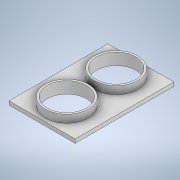
# Autodesk Inventor part: rinsing_station
Saved by Autodesk Inventor 2022 (Build 260153000, 153)
## iProperties
Created: 2022-05-04
Part Number: rinsing_station
Material: Generic
Document SubType Name: Modeling
Designer: cgbis
Density: 1 g/cm^3
Appearance: Default
Author: cgbis
Autodesk Inventor part; units mm, degrees
ref_plane "YZ Plane" through (0, 0, 0) normal (1, 0, 0) x (0, 1, 0)
ref_plane "XZ Plane" through (0, 0, 0) normal (0, 1, 0) x (-1, 0, 0)
ref_plane "XY Plane" through (0, 0, 0) normal (0, 0, 1) x (1, 0, 0)
sketch "Sketch1" plane through (0, 0, 0) normal (0, 1, 0) x (-1, 0, 0)
  point P0 (0, 0)
sketch "Sketch2" plane through (0, 0, 0) normal (0, 1, 0) x (-1, 0, 0)
  line L0 (0, 0) -> (85.5, 0)
  line L1 (85.5, 0) -> (85.5, -127.8)
  line L2 (85.5, -127.8) -> (0, -127.8)
  line L3 (0, -127.8) -> (0, 0)
  dimension "d0" = 85.5
  dimension "d1" = 127.8
  constraints: 8 end point, 2 parallel, 1 horizontal, 1 perpendicular
  measures "d0" distance of L1.end L2.end
  measures "d1" distance of L0.end L1.end
extrude "Extrusion1" add sketch "Sketch2" along normal blind 5
sketch "Sketch3" plane through (0, 5, 0) normal (0, 1, 0) x (1, 0, 0)
  line L0 (-85.5, 127.8) -> (-85.5, 0) projected
  line L1 (-85.5, 0) -> (0, 0)
  line L2 (0, 0) -> (0, 127.8)
  line L3 (0, 127.8) -> (-85.5, 127.8)
  line L4 (-85.5, 127.8) -> (-85.5, 0)
  line L5 (-2.4, 2.4) -> (-83.1, 2.4)
  line L6 (-83.1, 2.4) -> (-83.1, 125.4)
  line L7 (-83.1, 125.4) -> (-2.4, 125.4)
  line L8 (-2.4, 125.4) -> (-2.4, 2.4)
  dimension "d6" = 80.7
  dimension "d7" = 123
  constraints: 16 end point, 4 parallel, 2 horizontal, 2 perpendicular
  measures "d6" distance of L6.end L7.end
  measures "d7" distance of L5.end L6.end
extrude "Extrusion2" add sketch "Sketch3" along normal blind 120
sketch "Sketch4" plane through (0, 0, 0) normal (1, 0, 0) x (0, 0, -1)
  line L0 (10, 10) -> (117.8, 10)
  line L1 (117.8, 10) -> (117.8, 115)
  line L2 (117.8, 115) -> (10, 115)
  line L3 (10, 115) -> (10, 10)
  point P0 (0, 0)
  dimension "d10" = 107.8
  dimension "d11" = 105
  constraints: 8 end point, 2 parallel, 1 horizontal, 1 perpendicular
  measures "d10" distance of L2.end L1.end
  measures "d11" distance of L1.end L0.end
extrude "Extrusion3" cut sketch "Sketch4" against normal blind 500
sketch "Sketch5" plane through (0, 0, -127.8) normal (0, 0, -1) x (-1, 0, 0)
  line L0 (10, 10) -> (75.5, 10)
  line L1 (75.5, 10) -> (75.5, 115)
  line L2 (75.5, 115) -> (10, 115)
  line L3 (10, 115) -> (10, 10)
  point P0 (0, 0)
  dimension "d14" = 65.5
  dimension "d15" = 105
  constraints: 8 end point, 2 parallel, 1 horizontal, 1 perpendicular
  measures "d14" distance of L2.end L1.end
  measures "d15" distance of L1.end L0.end
extrude "Extrusion4" cut sketch "Sketch5" against normal blind 500
sketch "Sketch6" plane through (-85.5, 0, -127.8) normal (-1, 0, 0) x (0, 0, 1)
  line L0 (2.4, 125) -> (125.4, 125) projected
  line L1 (63.9, 125) -> (63.9, 0)
  line L2 (0, 0) -> (127.8, 0) projected
  line L3 (63.9, 125) -> (58.9, 125)
  line L4 (58.9, 125) -> (58.9, 0)
  line L5 (58.9, 0) -> (63.9, 0)
  line L6 (63.9, 0) -> (63.9, 125)
  line L7 (63.9, 125) -> (68.9, 125)
  line L8 (68.9, 125) -> (68.9, 0)
  line L9 (68.9, 0) -> (63.9, 0)
  line L10 (63.9, 0) -> (63.9, 125)
  dimension "d18" = 5
  dimension "d19" = 5
  constraints: 18 end point, 4 parallel, 2 horizontal, 2 midpoint, 2 perpendicular, 2 point on line
  measures "d18" distance of L5.end L4.end
  measures "d19" distance of L8.end L9.end
extrude "Extrusion5" add sketch "Sketch6" against normal blind 2.4
sketch "Sketch7" plane through (0, 0, 0) normal (1, 0, 0) x (0, 0, -1)
  line L0 (117.8, 115) -> (10, 115) projected
  line L1 (63.9, 115) -> (63.9, 10)
  line L2 (10, 10) -> (117.8, 10) projected
  line L3 (58.9, 10) -> (58.9, 115) projected
  line L4 (117.8, 10) -> (68.9, 10) projected
  line L5 (58.9, 115) -> (68.9, 115)
  line L6 (68.9, 115) -> (68.9, 10)
  line L7 (68.9, 10) -> (58.9, 10)
  line L8 (58.9, 10) -> (58.9, 115)
  point P0 (0, 0)
  constraints: 10 end point, 2 midpoint, 2 parallel, 1 horizontal, 1 perpendicular
extrude "Extrusion6" add sketch "Sketch7" against normal blind 2.4
sketch "Sketch8" plane through (0, 0, -127.8) normal (0, 0, -1) x (-1, 0, 0)
  line L0 (10, 100) -> (25, 115)
  line L1 (10, 115) -> (75.5, 115) projected
  line L2 (10, 100) -> (31.2132, 100) construction
  line L3 (75.5, 100) -> (60.5, 115)
  line L4 (75.5, 100) -> (96.7132, 100) construction
  line L5 (10, 10) -> (10, 115) projected
  line L6 (10, 25) -> (25, 10)
  line L7 (10, 10) -> (75.5, 10) projected
  line L8 (10, 25) -> (31.2132, 25) construction
  line L9 (75.5, 115) -> (75.5, 10) projected
  line L10 (75.5, 25) -> (60.5, 10)
  line L11 (10, 115) -> (75.5, 115)
  line L12 (75.5, 115) -> (75.5, 10)
  line L13 (75.5, 10) -> (10, 10)
  line L14 (10, 10) -> (10, 115)
  point P0 (0, 0)
  dimension "d24" = 45
  dimension "d25" = 135
  dimension "d26" = 45
  constraints: 22 end point, 6 point on line, 4 horizontal, 3 equal length, 2 parallel, 1 perpendicular
  measures "d24" angle of L2 L0
  measures "d25" angle of L4 L3
  measures "d26" angle of L6 L8
extrude "Extrusion7" add sketch "Sketch8" against normal blind 2.4 contours L5 L1 L0 | L6 L7 L5 | L1 L9 L3 | L10 L9 L7
sketch "Sketch9" plane through (-85.5, 0, 0) normal (0, 0, 1) x (1, 0, 0)
  line L0 (10, 25) -> (10, 100) projected
  line L1 (25, 115) -> (60.5, 115) projected
  line L2 (10, 100) -> (25, 115)
  line L3 (60.5, 115) -> (75.5, 100) projected
  line L4 (25, 115) -> (60.5, 115)
  line L5 (60.5, 115) -> (75.5, 100)
  line L6 (75.5, 100) -> (75.5, 25) projected
  line L7 (75.5, 100) -> (75.5, 25)
  line L8 (75.5, 25) -> (60.5, 10)
  line L9 (25, 10) -> (60.5, 10) projected
  line L10 (10, 25) -> (25, 10) projected
  line L11 (25, 10) -> (10, 25)
  line L12 (10, 25) -> (10, 100)
  line L13 (10, 115) -> (75.5, 115)
  line L14 (75.5, 115) -> (75.5, 10)
  line L15 (75.5, 10) -> (10, 10)
  line L16 (10, 10) -> (10, 115)
  point P0 (85.5, 0)
  point P1 (60.5, 10)
  constraints: 23 end point, 7 equal length, 2 horizontal, 1 perpendicular
extrude "Extrusion8" add sketch "Sketch9" against normal blind 2.4 contours L10 L15 L16 | L16 L13 L2 | L8 L14 L15 | L13 L14 L3
sketch "Sketch10" plane through (0, 0, 0) normal (1, 0, 0) x (0, 0, -1)
  line L0 (10, 115) -> (10, 10) projected
  line L1 (10, 100) -> (25, 115)
  line L2 (58.9, 115) -> (10, 115) projected
  line L3 (10, 100) -> (31.2132, 100) construction
  line L4 (58.9, 10) -> (58.9, 115) projected
  line L5 (58.9, 100) -> (43.9, 115)
  line L6 (58.9, 25) -> (43.9, 10)
  line L7 (10, 10) -> (58.9, 10) projected
  line L8 (10, 25) -> (25, 10)
  line L9 (68.9, 100) -> (83.9, 115)
  line L10 (68.9, 115) -> (117.8, 115) projected
  line L11 (68.9, 100) -> (90.1132, 100) construction
  line L12 (117.8, 115) -> (117.8, 10) projected
  line L13 (117.8, 100) -> (102.8, 115)
  line L14 (117.8, 25) -> (102.8, 10)
  line L15 (117.8, 10) -> (68.9, 10) projected
  line L16 (68.9, 25) -> (83.9, 10)
  line L17 (10, 115) -> (58.9, 115)
  line L18 (58.9, 115) -> (58.9, 10)
  line L19 (58.9, 10) -> (10, 10)
  line L20 (10, 10) -> (10, 115)
  line L21 (68.9, 115) -> (117.8, 115)
  line L22 (117.8, 115) -> (117.8, 10)
  line L23 (117.8, 10) -> (68.9, 10)
  line L24 (68.9, 10) -> (68.9, 115)
  point P0 (0, 0)
  dimension "d31" = 45
  dimension "d32" = 45
  constraints: 36 end point, 11 point on line, 6 perpendicular, 4 horizontal, 4 parallel, 2 equal length
  measures "d31" angle of L3 L1
  measures "d32" angle of L11 L9
extrude "Extrusion9" add sketch "Sketch10" against normal blind 2.4 contours L2 L1 L0 | L8 L7 L0 | L2 L4 L5 | L6 L4 L7 | L24 L10 L9 | L16 L15 L24 | L10 L12 L13 | L14 L12 L15
sketch "Sketch11" plane through (-85.5, 0, -127.8) normal (-1, 0, 0) x (0, 0, 1)
  line L0 (10, 100) -> (25, 115) projected
  line L1 (10, 100) -> (25, 115)
  line L2 (25, 115) -> (43.9, 115) projected
  line L3 (25, 115) -> (43.9, 115)
  line L4 (43.9, 115) -> (58.9, 100)
  line L5 (58.9, 100) -> (58.9, 25)
  line L6 (58.9, 25) -> (43.9, 10) projected
  line L7 (10, 10) -> (58.9, 10) projected
  line L8 (25, 10) -> (10, 25) projected
  line L9 (43.9, 10) -> (25, 10)
  line L10 (25, 10) -> (10, 25)
  line L11 (10, 25) -> (10, 100)
  line L12 (10, 115) -> (10, 10) projected
  line L13 (68.9, 25) -> (68.9, 100) projected
  line L14 (83.9, 115) -> (102.8, 115) projected
  line L15 (68.9, 100) -> (83.9, 115)
  line L16 (83.9, 115) -> (102.8, 115)
  line L17 (102.8, 115) -> (117.8, 100)
  line L18 (117.8, 25) -> (102.8, 10) projected
  line L19 (117.8, 100) -> (117.8, 25)
  line L20 (117.8, 25) -> (102.8, 10)
  line L21 (83.9, 10) -> (102.8, 10) projected
  line L22 (102.8, 10) -> (83.9, 10)
  line L23 (83.9, 10) -> (68.9, 25)
  line L24 (68.9, 25) -> (68.9, 100)
  line L25 (10, 115) -> (58.9, 115)
  line L26 (58.9, 115) -> (58.9, 10)
  line L27 (58.9, 10) -> (10, 10)
  line L28 (10, 10) -> (10, 115)
  line L29 (68.9, 115) -> (117.8, 115)
  line L30 (117.8, 115) -> (117.8, 10)
  line L31 (117.8, 10) -> (68.9, 10)
  line L32 (68.9, 10) -> (68.9, 115)
  point P0 (127.8, 0)
  constraints: 47 end point, 12 equal length, 8 perpendicular, 4 point on line, 2 horizontal
extrude "Extrusion10" add sketch "Sketch11" against normal blind 2.4 contours L12 L25 L0 | L8 L7 L12 | L25 L26 L4 | L6 L26 L7 | L23 L31 L32 | L32 L29 L15 | L18 L30 L31 | L29 L30 L17
sketch "Sketch12" plane through (0, 125, 0) normal (0, 1, 0) x (1, 0, 0)
  line L0 (-83.1, 125.4) -> (-2.4, 125.4) projected
  line L1 (-83.1, 125.4) -> (-83.1, 2.4) projected
  line L2 (-2.4, 125.4) -> (-83.1, 125.4)
  line L3 (-83.1, 125.4) -> (-83.1, 2.4)
  line L4 (-83.1, 2.4) -> (-2.4, 2.4)
  line L5 (-2.4, 2.4) -> (-2.4, 125.4)
  point P0 (0, 0)
  constraints: 8 end point, 2 parallel, 1 horizontal, 1 perpendicular
extrude "Extrusion11" add sketch "Sketch12" against normal blind 4.8
sketch "Sketch13" plane through (0, 125, 0) normal (0, 1, 0) x (1, 0, 0)
  line L0 (-2.4, 2.4) -> (-2.4, 125.4) projected
  line L1 (-83.1, 125.4) -> (-83.1, 2.4) projected
  line L2 (-2.4, 125.4) -> (-83.1, 125.4)
  line L3 (-83.1, 125.4) -> (-83.1, 2.4)
  line L4 (-83.1, 2.4) -> (-2.4, 2.4)
  line L5 (-2.4, 2.4) -> (-2.4, 125.4)
  point P0 (0, 0)
  constraints: 8 end point, 2 parallel, 1 horizontal, 1 perpendicular
extrude "Extrusion12" cut sketch "Sketch13" against normal blind 2.4
sketch "Sketch14" plane through (0, 122.6, 0) normal (0, 1, 0) x (1, 0, 0)
  line L0 (-80.1, 122.4) -> (-5.4, 122.4)
  line L1 (-5.4, 122.4) -> (-5.4, 5.4)
  line L2 (-5.4, 5.4) -> (-80.1, 5.4)
  line L3 (-80.1, 5.4) -> (-80.1, 122.4)
  point P0 (0, 0)
  dimension "d41" = 74.7
  dimension "d42" = 117
  constraints: 8 end point, 2 parallel, 1 horizontal, 1 perpendicular
  measures "d41" distance of L1.end L2.end
  measures "d42" distance of L0.end L1.end
extrude "Extrusion13" cut sketch "Sketch14" against normal blind 10
sketch "Sketch15" plane through (0, 0, 0) normal (1, 0, 0) x (0, 0, -1)
  line L0 (127.8, 0) -> (127.8, 125) projected
  line L1 (0, 125) -> (127.8, 125)
  line L2 (127.8, 125) -> (127.8, 119)
  line L3 (127.8, 119) -> (0, 119)
  line L4 (0, 119) -> (0, 125)
  line L5 (127.8, 125) -> (0, 125) projected
  line L6 (63.9, 125) -> (88.9, 125)
  line L7 (88.9, 125) -> (88.9, 119)
  line L8 (88.9, 119) -> (63.9, 119)
  line L9 (63.9, 119) -> (63.9, 125)
  line L10 (63.9, 125) -> (38.9, 125)
  line L11 (38.9, 125) -> (38.9, 119)
  line L12 (38.9, 119) -> (63.9, 119)
  line L13 (63.9, 119) -> (63.9, 125)
  point P0 (0, 0)
  dimension "d45" = 6
  dimension "d46" = 25
  dimension "d47" = 25
  constraints: 24 end point, 6 parallel, 3 horizontal, 3 perpendicular, 3 point on line, 1 midpoint
  measures "d45" distance of L1.end L2.end
  measures "d46" distance of L7.end L8.end
  measures "d47" distance of L12.end L11.end
extrude "Extrusion14" cut sketch "Sketch15" against normal blind 100 contours L3 L9 L1 L7 | L3 L11 L1 L9
sketch "Sketch16" plane through (0, 0, -127.8) normal (0, 0, -1) x (-1, 0, 0)
  line L0 (0, 125) -> (0, 119) projected
  line L1 (85.5, 0) -> (85.5, 125) projected
  line L2 (0, 125) -> (85.5, 125)
  line L3 (85.5, 125) -> (85.5, 119)
  line L4 (85.5, 119) -> (0, 119)
  line L5 (0, 119) -> (0, 125)
  line L6 (0, 125) -> (85.5, 125) projected
  line L7 (42.75, 125) -> (67.75, 125)
  line L8 (67.75, 125) -> (67.75, 119)
  line L9 (67.75, 119) -> (42.75, 119)
  line L10 (42.75, 119) -> (42.75, 125)
  line L11 (42.75, 125) -> (17.75, 125)
  line L12 (17.75, 125) -> (17.75, 119)
  line L13 (17.75, 119) -> (42.75, 119)
  line L14 (42.75, 119) -> (42.75, 125)
  point P0 (0, 0)
  dimension "d50" = 6
  dimension "d51" = 25
  dimension "d52" = 25
  constraints: 24 end point, 6 parallel, 3 horizontal, 3 perpendicular, 3 point on line, 1 midpoint
  measures "d50" distance of L2.end L3.end
  measures "d51" distance of L8.end L9.end
  measures "d52" distance of L13.end L12.end
extrude "Extrusion15" cut sketch "Sketch16" against normal blind 200 contours L2 L10 L4 L12 | L2 L8 L4 L10
sketch "Sketch17" plane through (-85.5, 0, 0) normal (0, 0, 1) x (1, 0, 0)
  line L0 (17.75, 119) -> (67.75, 119)
  line L1 (67.75, 119) -> (67.75, 118)
  line L2 (67.75, 118) -> (17.75, 118)
  line L3 (17.75, 118) -> (17.75, 119)
  point P0 (85.5, 0)
  dimension "d55" = 1
  constraints: 8 end point, 2 parallel, 1 horizontal, 1 perpendicular
  measures "d55" distance of L0.end L1.end
extrude "Extrusion16" cut sketch "Sketch17" against normal blind 200
sketch "Sketch18" plane through (0, 0, 0) normal (1, 0, 0) x (0, 0, -1)
  line L0 (38.9, 119) -> (38.9, 120.2) projected
  line L1 (38.9, 119) -> (88.9, 119)
  line L2 (88.9, 119) -> (88.9, 118)
  line L3 (88.9, 118) -> (38.9, 118)
  line L4 (38.9, 118) -> (38.9, 119)
  point P0 (0, 0)
  dimension "d58" = 1
  constraints: 8 end point, 2 parallel, 1 horizontal, 1 perpendicular
  measures "d58" distance of L1.end L2.end
extrude "Extrusion17" cut sketch "Sketch18" against normal blind 200
sketch "Sketch19" plane through (0, 0, -127.8) normal (0, 0, -1) x (-1, 0, 0)
  line L0 (17.75, 118) -> (67.75, 118) projected
  line L1 (17.75, 118) -> (67.75, 118)
  line L2 (67.75, 118) -> (67.75, 112)
  line L3 (67.75, 112) -> (17.75, 112)
  line L4 (17.75, 112) -> (17.75, 118)
  point P0 (0, 0)
  dimension "d61" = 50
  dimension "d62" = 6
  constraints: 8 end point, 2 parallel, 1 horizontal, 1 perpendicular
  measures "d61" distance of L2.end L3.end
  measures "d62" distance of L1.end L2.end
extrude "Extrusion18" add sketch "Sketch19" against normal blind 2.4
sketch "Sketch20" plane through (-85.5, 0, -127.8) normal (-1, 0, 0) x (0, 0, 1)
  line L0 (2.4, 118) -> (0, 118) projected
  line L1 (127.8, 100) -> (127.8, 115) projected
  line L2 (0, 118) -> (127.8, 118)
  line L3 (127.8, 118) -> (127.8, 112)
  line L4 (127.8, 112) -> (0, 112)
  line L5 (0, 112) -> (0, 118)
  point P0 (127.8, 0)
  dimension "d65" = 6
  constraints: 8 end point, 2 parallel, 1 horizontal, 1 perpendicular, 1 point on line
  measures "d65" distance of L2.end L3.end
extrude "Extrusion19" add sketch "Sketch20" against normal blind 2.4
sketch "Sketch21" plane through (-85.5, 0, 0) normal (0, 0, 1) x (1, 0, 0)
  line L0 (17.75, 118) -> (67.75, 118) projected
  line L1 (17.75, 118) -> (67.75, 118)
  line L2 (67.75, 118) -> (67.75, 112)
  line L3 (67.75, 112) -> (17.75, 112)
  line L4 (17.75, 112) -> (17.75, 118)
  point P0 (85.5, 0)
  dimension "d68" = 6
  constraints: 8 end point, 2 parallel, 1 horizontal, 1 perpendicular
  measures "d68" distance of L1.end L2.end
extrude "Extrusion20" add sketch "Sketch21" against normal blind 2.4
sketch "Sketch22" plane through (0, 0, 0) normal (1, 0, 0) x (0, 0, -1)
  line L0 (127.8, 0) -> (127.8, 125) projected
  line L1 (0, 118) -> (127.8, 118)
  line L2 (127.8, 118) -> (127.8, 112)
  line L3 (127.8, 112) -> (0, 112)
  line L4 (0, 112) -> (0, 118)
  point P0 (0, 0)
  dimension "d71" = 6
  constraints: 8 end point, 2 parallel, 1 horizontal, 1 perpendicular, 1 point on line
  measures "d71" distance of L1.end L2.end
extrude "Extrusion21" add sketch "Sketch22" against normal blind 2.4
sketch "Sketch23" plane through (0, 125, 0) normal (0, 1, 0) x (1, 0, 0)
  line L0 (-85.5, 127.8) -> (-85.5, 0) projected
  line L1 (-85.5, 127.8) -> (0, 127.8)
  line L2 (0, 127.8) -> (0, 0)
  line L3 (0, 0) -> (-85.5, 0)
  line L4 (-85.5, 0) -> (-85.5, 127.8)
  constraints: 8 end point, 2 parallel, 1 horizontal, 1 perpendicular
extrude "Extrusion22" cut sketch "Sketch23" against normal blind 120
sketch "Sketch24" plane through (0, 5, 0) normal (0, 1, 0) x (1, 0, 0)
  line L0 (0, 127.8) -> (-85.5, 127.8) projected
  line L1 (-42.75, 127.8) -> (-42.75, 0)
  line L2 (-85.5, 0) -> (0, 0) projected
  line L3 (-85.5, 127.8) -> (-85.5, 0) projected
  line L4 (-85.5, 63.9) -> (0, 63.9)
  line L5 (0, 0) -> (0, 127.8) projected
  line L6 (-42.75, 63.9) -> (-36.25, 63.9)
  line L7 (-36.25, 63.9) -> (-36.25, 70.4)
  line L8 (-36.25, 70.4) -> (-42.75, 70.4)
  line L9 (-42.75, 70.4) -> (-42.75, 63.9)
  line L10 (-36.25, 70.4) -> (-49.25, 70.4)
  line L11 (-49.25, 70.4) -> (-49.25, 57.4)
  line L12 (-49.25, 57.4) -> (-36.25, 57.4)
  line L13 (-36.25, 57.4) -> (-36.25, 70.4)
  line L14 (-42.75, 63.9) -> (-34.75, 63.9)
  line L15 (-34.75, 63.9) -> (-34.75, 71.9)
  line L16 (-34.75, 71.9) -> (-42.75, 71.9)
  line L17 (-42.75, 71.9) -> (-42.75, 63.9)
  line L18 (-34.75, 71.9) -> (-50.75, 71.9)
  line L19 (-50.75, 71.9) -> (-50.75, 55.9)
  line L20 (-50.75, 55.9) -> (-34.75, 55.9)
  line L21 (-34.75, 55.9) -> (-34.75, 71.9)
  dimension "d76" = 6.5
  dimension "d77" = 6.5
  dimension "d78" = 13
  dimension "d79" = 13
  dimension "d80" = 8
  dimension "d81" = 8
  dimension "d82" = 16
  dimension "d83" = 16
  constraints: 36 end point, 8 parallel, 5 midpoint, 4 horizontal, 4 perpendicular
  measures "d76" distance of L8.end L7.end
  measures "d77" distance of L7.end L6.end
  measures "d78" distance of L12.end L11.end
  measures "d79" distance of L11.end L10.end
  measures "d80" distance of L16.end L15.end
  measures "d81" distance of L15.end L14.end
  measures "d82" distance of L20.end L19.end
  measures "d83" distance of L19.end L18.end
extrude "Extrusion23" add sketch "Sketch24" along normal blind 25 contours L16 L15 L4 L7 L8 L1 | L1 L10 L11 L4 L19 L18 | L21 L20 L1 L12 L13 L4 | L4 L11 L12 L1 L20 L19
sketch "Sketch26" plane through (0, 30, 0) normal (0, 1, 0) x (1, 0, 0)
  line L0 (-60.75, 81.9) -> (-60.75, 68.9) projected
  line L1 (-24.75, 45.9) -> (-37.75, 45.9) projected
  line L2 (-60.75, 81.9) -> (-24.75, 81.9)
  line L3 (-24.75, 81.9) -> (-24.75, 45.9)
  line L4 (-24.75, 45.9) -> (-60.75, 45.9)
  line L5 (-60.75, 45.9) -> (-60.75, 81.9)
  point P0 (0, 0)
  constraints: 8 end point, 2 parallel, 1 horizontal, 1 perpendicular
extrude "Extrusion25" cut sketch "Sketch26" against normal blind 25
sketch "Sketch27" plane through (0, 5, 0) normal (0, 1, 0) x (1, 0, 0)
  line L0 (0, 127.8) -> (-85.5, 127.8) projected
  line L1 (-85.5, 127.8) -> (0, 127.8)
  line L2 (0, 127.8) -> (0, 0)
  line L3 (0, 0) -> (-85.5, 0)
  line L4 (-85.5, 0) -> (-85.5, 127.8)
  line L5 (-42.75, 127.8) -> (-42.75, 0)
  line L6 (0, 0) -> (0, 127.8) projected
  line L7 (-85.5, 127.8) -> (0, 127.8)
  line L8 (0, 127.8) -> (0, 117.8)
  line L9 (0, 117.8) -> (-85.5, 117.8)
  line L10 (-85.5, 117.8) -> (-85.5, 127.8)
  line L11 (-85.5, 127.8) -> (-85.5, 0) projected
  line L12 (0, 117.8) -> (-85.5, 117.8)
  line L13 (-85.5, 117.8) -> (-85.5, 97.8)
  line L14 (-85.5, 97.8) -> (0, 97.8)
  line L15 (0, 97.8) -> (0, 117.8)
  line L16 (-85.5, 97.8) -> (0, 97.8)
  line L17 (0, 97.8) -> (0, 77.8)
  line L18 (0, 77.8) -> (-85.5, 77.8)
  line L19 (-85.5, 77.8) -> (-85.5, 97.8)
  line L20 (-85.5, 77.8) -> (0, 77.8)
  line L21 (0, 77.8) -> (0, 57.8)
  line L22 (0, 57.8) -> (-85.5, 57.8)
  line L23 (-85.5, 57.8) -> (-85.5, 77.8)
  line L24 (-85.5, 57.8) -> (0, 57.8)
  line L25 (0, 57.8) -> (0, 37.8)
  line L26 (0, 37.8) -> (-85.5, 37.8)
  line L27 (-85.5, 37.8) -> (-85.5, 57.8)
  line L28 (-85.5, 37.8) -> (0, 37.8)
  line L29 (0, 37.8) -> (0, 17.8)
  line L30 (0, 17.8) -> (-85.5, 17.8)
  line L31 (-85.5, 17.8) -> (-85.5, 37.8)
  line L32 (-85.5, 127.8) -> (-42.75, 127.8)
  line L33 (0, 127.8) -> (-42.75, 127.8)
  line L34 (-64.125, 127.8) -> (-64.125, 0)
  line L35 (-85.5, 0) -> (0, 0) projected
  line L36 (-21.375, 127.8) -> (-21.375, 0)
  line L37 (-62.625, 127.8) -> (-65.625, 127.8)
  line L38 (-65.625, 127.8) -> (-65.625, 0)
  line L39 (-65.625, 0) -> (-62.625, 0)
  line L40 (-62.625, 0) -> (-62.625, 127.8)
  line L41 (-41.25, 127.8) -> (-44.25, 127.8)
  line L42 (-44.25, 127.8) -> (-44.25, 0)
  line L43 (-44.25, 0) -> (-41.25, 0)
  line L44 (-41.25, 0) -> (-41.25, 127.8)
  line L45 (-19.875, 127.8) -> (-22.875, 127.8)
  line L46 (-22.875, 127.8) -> (-22.875, 0)
  line L47 (-22.875, 0) -> (-19.875, 0)
  line L48 (-19.875, 0) -> (-19.875, 127.8)
  line L49 (-85.5, 117.8) -> (0, 117.8)
  line L50 (0, 117.8) -> (0, 120.8)
  line L51 (0, 120.8) -> (-85.5, 120.8)
  line L52 (-85.5, 120.8) -> (-85.5, 117.8)
  line L53 (-85.5, 120.8) -> (0, 120.8)
  line L54 (0, 120.8) -> (0, 114.8)
  line L55 (0, 114.8) -> (-85.5, 114.8)
  line L56 (-85.5, 114.8) -> (-85.5, 120.8)
  line L57 (-85.5, 97.8) -> (0, 97.8)
  line L58 (0, 97.8) -> (0, 100.8)
  line L59 (0, 100.8) -> (-85.5, 100.8)
  line L60 (-85.5, 100.8) -> (-85.5, 97.8)
  line L61 (0, 97.8) -> (-85.5, 97.8)
  line L62 (-85.5, 97.8) -> (-85.5, 94.8)
  line L63 (-85.5, 94.8) -> (0, 94.8)
  line L64 (0, 94.8) -> (0, 97.8)
  line L65 (-85.5, 77.8) -> (0, 77.8)
  line L66 (0, 77.8) -> (0, 80.8)
  line L67 (0, 80.8) -> (-85.5, 80.8)
  line L68 (-85.5, 80.8) -> (-85.5, 77.8)
  line L69 (0, 80.8) -> (-85.5, 80.8)
  line L70 (-85.5, 80.8) -> (-85.5, 74.8)
  line L71 (-85.5, 74.8) -> (0, 74.8)
  line L72 (0, 74.8) -> (0, 80.8)
  line L73 (-85.5, 57.8) -> (0, 57.8)
  line L74 (0, 57.8) -> (0, 60.8)
  line L75 (0, 60.8) -> (-85.5, 60.8)
  line L76 (-85.5, 60.8) -> (-85.5, 57.8)
  line L77 (0, 60.8) -> (-85.5, 60.8)
  line L78 (-85.5, 60.8) -> (-85.5, 54.8)
  line L79 (-85.5, 54.8) -> (0, 54.8)
  line L80 (0, 54.8) -> (0, 60.8)
  line L81 (-85.5, 37.8) -> (0, 37.8)
  line L82 (0, 37.8) -> (0, 40.8)
  line L83 (0, 40.8) -> (-85.5, 40.8)
  line L84 (-85.5, 40.8) -> (-85.5, 37.8)
  line L85 (-85.5, 40.8) -> (0, 40.8)
  line L86 (0, 40.8) -> (0, 34.8)
  line L87 (0, 34.8) -> (-85.5, 34.8)
  line L88 (-85.5, 34.8) -> (-85.5, 40.8)
  line L89 (-85.5, 17.8) -> (0, 17.8)
  line L90 (0, 17.8) -> (0, 20.8)
  line L91 (0, 20.8) -> (-85.5, 20.8)
  line L92 (-85.5, 20.8) -> (-85.5, 17.8)
  line L93 (0, 20.8) -> (-85.5, 20.8)
  line L94 (-85.5, 20.8) -> (-85.5, 14.8)
  line L95 (-85.5, 14.8) -> (0, 14.8)
  line L96 (0, 14.8) -> (0, 20.8)
  point P0 (-22.875, 20.8)
  point P1 (-22.875, 17.8)
  point P2 (-19.875, 17.8)
  point P3 (-19.875, 20.8)
  point P4 (-44.25, 20.8)
  point P5 (-44.25, 14.8)
  point P6 (-41.25, 14.8)
  point P7 (-41.25, 20.8)
  point P8 (-65.625, 20.8)
  point P9 (-65.625, 14.8)
  point P10 (-62.625, 14.8)
  point P11 (-62.625, 20.8)
  point P12 (-19.875, 40.8)
  point P13 (-22.875, 40.8)
  point P14 (-22.875, 34.8)
  point P15 (-19.875, 34.8)
  point P16 (-41.25, 40.8)
  point P17 (-44.25, 40.8)
  point P18 (-44.25, 34.8)
  point P19 (-41.25, 34.8)
  point P20 (-62.625, 40.8)
  point P21 (-65.625, 40.8)
  point P22 (-65.625, 34.8)
  point P23 (-62.625, 34.8)
  point P24 (-22.875, 60.8)
  point P25 (-22.875, 54.8)
  point P26 (-19.875, 54.8)
  point P27 (-19.875, 60.8)
  point P28 (-44.25, 60.8)
  point P29 (-44.25, 54.8)
  point P30 (-41.25, 54.8)
  point P31 (-41.25, 60.8)
  point P32 (-65.625, 60.8)
  point P33 (-65.625, 54.8)
  point P34 (-62.625, 54.8)
  point P35 (-62.625, 60.8)
  point P36 (-44.25, 80.8)
  point P37 (-44.25, 74.8)
  point P38 (-41.25, 74.8)
  point P39 (-41.25, 80.8)
  point P40 (-62.625, 80.8)
  point P41 (-65.625, 80.8)
  point P42 (-65.625, 74.8)
  point P43 (-62.625, 74.8)
  point P44 (-19.875, 80.8)
  point P45 (-22.875, 80.8)
  point P46 (-22.875, 74.8)
  point P47 (-19.875, 74.8)
  point P48 (-19.875, 100.8)
  point P49 (-22.875, 100.8)
  point P50 (-22.875, 94.8)
  point P51 (-19.875, 94.8)
  point P52 (-41.25, 94.8)
  point P53 (-41.25, 100.8)
  point P54 (-44.25, 100.8)
  point P55 (-44.25, 94.8)
  point P56 (-65.625, 100.8)
  point P57 (-65.625, 94.8)
  point P58 (-62.625, 94.8)
  point P59 (-62.625, 100.8)
  point P60 (-19.875, 120.8)
  point P61 (-22.875, 120.8)
  point P62 (-22.875, 114.8)
  point P63 (-19.875, 114.8)
  point P64 (-41.25, 120.8)
  point P65 (-44.25, 120.8)
  point P66 (-44.25, 114.8)
  point P67 (-41.25, 114.8)
  point P68 (-62.625, 120.8)
  point P69 (-65.625, 120.8)
  point P70 (-65.625, 114.8)
  point P71 (-62.625, 114.8)
  dimension "d100" = 10
  dimension "d101" = 20
  dimension "d102" = 20
  dimension "d103" = 20
  dimension "d104" = 20
  dimension "d105" = 20
  dimension "d106" = 3
  dimension "d107" = 3
  dimension "d108" = 3
  dimension "d109" = 3
  dimension "d110" = 6
  dimension "d111" = 3
  dimension "d112" = 3
  dimension "d113" = 3
  dimension "d114" = 6
  dimension "d115" = 3
  dimension "d116" = 85.5
  dimension "d117" = 6
  dimension "d118" = 3
  dimension "d119" = 6
  dimension "d120" = 3
  dimension "d121" = 6
  constraints: 186 end point, 44 parallel, 25 point on line, 24 perpendicular, 22 horizontal, 4 midpoint, 2 collinear
  measures "d100" distance of L7.end L8.end
  measures "d101" distance of L13.end L12.end
  measures "d102" distance of L16.end L17.end
  measures "d103" distance of L20.end L21.end
  measures "d104" distance of L24.end L25.end
  measures "d105" distance of L28.end L29.end
  measures "d106" distance of L39.end L38.end
  measures "d107" distance of L43.end L42.end
  measures "d108" distance of L47.end L46.end
  measures "d109" distance of L50.end L49.end
  measures "d110" distance of L53.end L54.end
  measures "d111" distance of L58.end L57.end
  measures "d112" distance of L62.end L61.end
  measures "d113" distance of L66.end L65.end
  measures "d114" distance of L70.end L69.end
  measures "d115" distance of L74.end L73.end
  measures "d116" distance of L79.end L78.end
  measures "d117" distance of L78.end L77.end
  measures "d118" distance of L82.end L81.end
  measures "d119" distance of L85.end L86.end
  measures "d120" distance of L90.end L89.end
  measures "d121" distance of L94.end L93.end
extrude "Extrusion26" cut sketch "Sketch27" against normal blind 5 contours L48 L9 L36 L51 | L36 L9 L46 L51 | L48 L55 L36 L9 | L36 L55 L46 L9 | L44 L9 L5 L51 | L48 L14 L36 L59 | L5 L9 L42 L51 | L44 L55 L5 L9 | L36 L14 L46 L59 | L48 L63 L36 L14 | L5 L55 L42 L9 | L36 L63 L46 L14 | L40 L9 L34 L51 | L44 L14 L5 L59 | L48 L18 L36 L67 | L34 L9 L38 L51 | L40 L55 L34 L9 | L5 L14 L42 L59 | L44 L63 L5 L14 | L36 L18 L46 L67 | L48 L71 L36 L18 | L34 L55 L38 L9 | L5 L63 L42 L14 | L36 L71 L46 L18 | L40 L14 L34 L59 | L44 L18 L5 L67 | L48 L22 L36 L75 | L34 L14 L38 L59 | L40 L63 L34 L14 | L5 L18 L42 L67 | L44 L71 L5 L18 | L36 L22 L46 L75 | L48 L79 L36 L22 | L34 L63 L38 L14 | L5 L71 L42 L18 | L36 L79 L46 L22 | L40 L18 L34 L67 | L44 L22 L5 L75 | L48 L26 L36 L83 | L34 L18 L38 L67 | L40 L71 L34 L18 | L5 L22 L42 L75 | L44 L79 L5 L22 | L36 L26 L46 L83 | L48 L87 L36 L26 | L34 L71 L38 L18 | L5 L79 L42 L22 | L36 L87 L46 L26 | L40 L22 L34 L75 | L44 L26 L5 L83 | L48 L30 L36 L91 | L34 L22 L38 L75 | L40 L79 L34 L22 | L5 L26 L42 L83 | L44 L87 L5 L26 | L36 L30 L46 L91 | L34 L79 L38 L22 | L5 L87 L42 L26 | L40 L26 L34 L83 | L44 L30 L5 L91 | L34 L26 L38 L83 | L40 L87 L34 L26 | L5 L30 L42 L91 | L44 L95 L5 L30 | L34 L87 L38 L26 | L5 L95 L42 L30 | L40 L30 L34 L91 | L34 L30 L38 L91 | L40 L95 L34 L30 | L34 L95 L38 L30
sketch "Sketch28" plane through (0, 5, 0) normal (0, 1, 0) x (1, 0, 0)
  line L0 (-22.875, 17.8) -> (-19.875, 17.8) projected
  line L1 (-19.875, 17.8) -> (-22.875, 17.8)
  line L2 (-22.875, 17.8) -> (-22.875, 14.8)
  line L3 (-22.875, 14.8) -> (-19.875, 14.8)
  line L4 (-19.875, 14.8) -> (-19.875, 17.8)
  point P0 (0, 0)
  dimension "d124" = 3
  dimension "d125" = 3
  constraints: 8 end point, 2 parallel, 1 horizontal, 1 perpendicular
  measures "d124" distance of L3.end L2.end
  measures "d125" distance of L2.end L1.end
extrude "Extrusion27" cut sketch "Sketch28" against normal blind 5
sketch "Sketch29" plane through (0, 5, 0) normal (0, 1, 0) x (1, 0, 0)
  line L0 (-22.875, 14.8) -> (-22.875, 20.8) projected
  line L1 (-22.875, 20.8) -> (-19.875, 20.8) projected
  line L2 (-19.875, 20.8) -> (-19.875, 14.8) projected
  line L3 (-19.875, 14.8) -> (-22.875, 14.8) projected
  line L4 (-19.875, 114.8) -> (-22.875, 114.8) projected
  line L5 (-22.875, 114.8) -> (-22.875, 120.8) projected
  line L6 (-22.875, 120.8) -> (-19.875, 120.8) projected
  line L7 (-19.875, 120.8) -> (-19.875, 114.8) projected
  line L8 (-19.875, 74.8) -> (-22.875, 74.8) projected
  line L9 (-22.875, 74.8) -> (-22.875, 80.8) projected
  line L10 (-22.875, 80.8) -> (-19.875, 80.8) projected
  line L11 (-19.875, 80.8) -> (-19.875, 74.8) projected
  line L12 (-41.25, 54.8) -> (-44.25, 54.8) projected
  line L13 (-44.25, 54.8) -> (-44.25, 60.8) projected
  line L14 (-44.25, 60.8) -> (-41.25, 60.8) projected
  line L15 (-41.25, 60.8) -> (-41.25, 54.8) projected
  line L16 (-19.875, 34.8) -> (-22.875, 34.8) projected
  line L17 (-22.875, 34.8) -> (-22.875, 40.8) projected
  line L18 (-22.875, 40.8) -> (-19.875, 40.8) projected
  line L19 (-19.875, 40.8) -> (-19.875, 34.8) projected
  line L20 (-41.25, 34.8) -> (-44.25, 34.8) projected
  line L21 (-44.25, 34.8) -> (-44.25, 40.8) projected
  line L22 (-44.25, 40.8) -> (-41.25, 40.8) projected
  line L23 (-41.25, 40.8) -> (-41.25, 34.8) projected
  line L24 (-62.625, 54.8) -> (-65.625, 54.8) projected
  line L25 (-65.625, 54.8) -> (-65.625, 60.8) projected
  line L26 (-65.625, 60.8) -> (-62.625, 60.8) projected
  line L27 (-62.625, 60.8) -> (-62.625, 54.8) projected
  line L28 (-19.875, 94.8) -> (-22.875, 94.8) projected
  line L29 (-22.875, 94.8) -> (-22.875, 100.8) projected
  line L30 (-22.875, 100.8) -> (-19.875, 100.8) projected
  line L31 (-19.875, 100.8) -> (-19.875, 94.8) projected
  line L32 (-41.25, 114.8) -> (-44.25, 114.8) projected
  line L33 (-44.25, 114.8) -> (-44.25, 120.8) projected
  line L34 (-44.25, 120.8) -> (-41.25, 120.8) projected
  line L35 (-41.25, 120.8) -> (-41.25, 114.8) projected
  line L36 (-62.625, 94.8) -> (-65.625, 94.8) projected
  line L37 (-65.625, 94.8) -> (-65.625, 100.8) projected
  line L38 (-65.625, 100.8) -> (-62.625, 100.8) projected
  line L39 (-62.625, 100.8) -> (-62.625, 94.8) projected
  line L40 (-62.625, 74.8) -> (-65.625, 74.8) projected
  line L41 (-65.625, 74.8) -> (-65.625, 80.8) projected
  line L42 (-65.625, 80.8) -> (-62.625, 80.8) projected
  line L43 (-62.625, 80.8) -> (-62.625, 74.8) projected
  line L44 (-19.875, 54.8) -> (-22.875, 54.8) projected
  line L45 (-22.875, 54.8) -> (-22.875, 60.8) projected
  line L46 (-22.875, 60.8) -> (-19.875, 60.8) projected
  line L47 (-19.875, 60.8) -> (-19.875, 54.8) projected
  line L48 (-62.625, 14.8) -> (-65.625, 14.8) projected
  line L49 (-65.625, 14.8) -> (-65.625, 20.8) projected
  line L50 (-65.625, 20.8) -> (-62.625, 20.8) projected
  line L51 (-62.625, 20.8) -> (-62.625, 14.8) projected
  line L52 (-41.25, 14.8) -> (-44.25, 14.8) projected
  line L53 (-44.25, 14.8) -> (-44.25, 20.8) projected
  line L54 (-44.25, 20.8) -> (-41.25, 20.8) projected
  line L55 (-41.25, 20.8) -> (-41.25, 14.8) projected
  line L56 (-62.625, 34.8) -> (-65.625, 34.8) projected
  line L57 (-65.625, 34.8) -> (-65.625, 40.8) projected
  line L58 (-65.625, 40.8) -> (-62.625, 40.8) projected
  line L59 (-62.625, 40.8) -> (-62.625, 34.8) projected
  line L60 (-41.25, 74.8) -> (-44.25, 74.8) projected
  line L61 (-44.25, 74.8) -> (-44.25, 80.8) projected
  line L62 (-44.25, 80.8) -> (-41.25, 80.8) projected
  line L63 (-41.25, 80.8) -> (-41.25, 74.8) projected
  line L64 (-44.25, 100.8) -> (-41.25, 100.8) projected
  line L65 (-41.25, 100.8) -> (-41.25, 94.8) projected
  line L66 (-41.25, 94.8) -> (-44.25, 94.8) projected
  line L67 (-44.25, 94.8) -> (-44.25, 100.8) projected
  line L68 (-62.625, 114.8) -> (-65.625, 114.8) projected
  line L69 (-65.625, 114.8) -> (-65.625, 120.8) projected
  line L70 (-65.625, 120.8) -> (-62.625, 120.8) projected
  line L71 (-62.625, 120.8) -> (-62.625, 114.8) projected
  line L72 (0, 127.8) -> (0, 0) projected
  line L73 (-85.5, 127.8) -> (0, 127.8) projected
  line L74 (-85.5, 0) -> (-85.5, 127.8) projected
  line L75 (0, 0) -> (-85.5, 0) projected
extrude "Extrusion28" add sketch "Sketch29" along normal blind 10
sketch "Sketch30" plane through (-85.5, 0, 0) normal (0, 0, 1) x (1, 0, 0)
  line L0 (0, 0) -> (0, 15) projected
  line L1 (0, 0) -> (85.5, 0) projected
  line L2 (85.5, 0) -> (85.5, 15) projected
  line L3 (0, 15) -> (85.5, 15) projected
extrude "Extrusion29" cut sketch "Sketch30" against normal blind 3.9
sketch "Sketch31" plane through (0, 0, -127.8) normal (0, 0, -1) x (-1, 0, 0)
  line L0 (0, 0) -> (0, 15) projected
  line L1 (0, 0) -> (85.5, 0) projected
  line L2 (85.5, 0) -> (85.5, 15) projected
  line L3 (0, 15) -> (85.5, 15) projected
extrude "Extrusion30" add sketch "Sketch31" along normal blind 3.9
sketch "Sketch32" plane through (0, 15, 0) normal (0, 1, 0) x (1, 0, 0)
  line L0 (-85.5, 3.9) -> (-85.5, 131.7) projected
  line L1 (-85.5, 3.9) -> (0, 3.9) projected
  line L2 (-85.5, 131.7) -> (-75.5, 131.7)
  line L3 (-75.5, 131.7) -> (-75.5, 3.9)
  line L4 (-75.5, 3.9) -> (-85.5, 3.9)
  line L5 (-85.5, 3.9) -> (-85.5, 131.7)
  line L6 (0, 3.9) -> (0, 131.7) projected
  line L7 (0, 131.7) -> (-10, 131.7)
  line L8 (-10, 131.7) -> (-10, 3.9)
  line L9 (-10, 3.9) -> (0, 3.9)
  line L10 (0, 3.9) -> (0, 131.7)
  point P0 (0, 0)
  point P1 (-10, 3.9)
  dimension "d140" = 10
  dimension "d141" = 10
  constraints: 16 end point, 4 parallel, 2 horizontal, 2 perpendicular, 2 point on line
  measures "d140" distance of L3.end L4.end
  measures "d141" distance of L9.end L8.end
extrude "Extrusion31" cut sketch "Sketch32" against normal blind 10
sketch "Sketch33" plane through (0, 15, 0) normal (0, 1, 0) x (1, 0, 0)
  line L0 (-65.625, 120.8) -> (-65.625, 114.8) projected
  line L1 (-65.625, 120.8) -> (-62.625, 120.8)
  line L2 (-62.625, 120.8) -> (-62.625, 122.8)
  line L3 (-62.625, 122.8) -> (-65.625, 122.8)
  line L4 (-65.625, 122.8) -> (-65.625, 120.8)
  line L5 (-65.625, 114.8) -> (-62.625, 114.8) projected
  line L6 (-65.625, 114.8) -> (-62.625, 114.8)
  line L7 (-62.625, 114.8) -> (-62.625, 112.8)
  line L8 (-62.625, 112.8) -> (-65.625, 112.8)
  line L9 (-65.625, 112.8) -> (-65.625, 114.8)
  line L10 (-41.25, 120.8) -> (-44.25, 120.8) projected
  line L11 (-44.25, 120.8) -> (-41.25, 120.8)
  line L12 (-41.25, 120.8) -> (-41.25, 122.8)
  line L13 (-41.25, 122.8) -> (-44.25, 122.8)
  line L14 (-44.25, 122.8) -> (-44.25, 120.8)
  line L15 (-19.875, 120.8) -> (-22.875, 120.8) projected
  line L16 (-22.875, 120.8) -> (-19.875, 120.8)
  line L17 (-19.875, 120.8) -> (-19.875, 122.8)
  line L18 (-19.875, 122.8) -> (-22.875, 122.8)
  line L19 (-22.875, 122.8) -> (-22.875, 120.8)
  line L20 (-44.25, 114.8) -> (-41.25, 114.8)
  line L21 (-41.25, 114.8) -> (-41.25, 112.8)
  line L22 (-41.25, 112.8) -> (-44.25, 112.8)
  line L23 (-44.25, 112.8) -> (-44.25, 114.8)
  line L24 (-22.875, 114.8) -> (-19.875, 114.8) projected
  line L25 (-22.875, 114.8) -> (-19.875, 114.8)
  line L26 (-19.875, 114.8) -> (-19.875, 112.8)
  line L27 (-19.875, 112.8) -> (-22.875, 112.8)
  line L28 (-22.875, 112.8) -> (-22.875, 114.8)
  line L29 (-62.625, 100.8) -> (-65.625, 100.8) projected
  line L30 (-65.625, 100.8) -> (-62.625, 100.8)
  line L31 (-62.625, 100.8) -> (-62.625, 102.8)
  line L32 (-62.625, 102.8) -> (-65.625, 102.8)
  line L33 (-65.625, 102.8) -> (-65.625, 100.8)
  line L34 (-65.625, 94.8) -> (-62.625, 94.8) projected
  line L35 (-65.625, 94.8) -> (-62.625, 94.8)
  line L36 (-62.625, 94.8) -> (-62.625, 92.8)
  line L37 (-62.625, 92.8) -> (-65.625, 92.8)
  line L38 (-65.625, 92.8) -> (-65.625, 94.8)
  line L39 (-44.25, 100.8) -> (-44.25, 94.8) projected
  line L40 (-44.25, 100.8) -> (-41.25, 100.8)
  line L41 (-41.25, 100.8) -> (-41.25, 102.8)
  line L42 (-41.25, 102.8) -> (-44.25, 102.8)
  line L43 (-44.25, 102.8) -> (-44.25, 100.8)
  line L44 (-44.25, 94.8) -> (-41.25, 94.8)
  line L45 (-41.25, 94.8) -> (-41.25, 92.8)
  line L46 (-41.25, 92.8) -> (-44.25, 92.8)
  line L47 (-44.25, 92.8) -> (-44.25, 94.8)
  line L48 (-22.875, 100.8) -> (-22.875, 94.8) projected
  line L49 (-22.875, 100.8) -> (-19.875, 100.8)
  line L50 (-19.875, 100.8) -> (-19.875, 102.8)
  line L51 (-19.875, 102.8) -> (-22.875, 102.8)
  line L52 (-22.875, 102.8) -> (-22.875, 100.8)
  line L53 (-22.875, 94.8) -> (-19.875, 94.8)
  line L54 (-19.875, 94.8) -> (-19.875, 92.8)
  line L55 (-19.875, 92.8) -> (-22.875, 92.8)
  line L56 (-22.875, 92.8) -> (-22.875, 94.8)
  line L57 (-65.625, 80.8) -> (-65.625, 74.8) projected
  line L58 (-65.625, 80.8) -> (-62.625, 80.8)
  line L59 (-62.625, 80.8) -> (-62.625, 82.8)
  line L60 (-62.625, 82.8) -> (-65.625, 82.8)
  line L61 (-65.625, 82.8) -> (-65.625, 80.8)
  line L62 (-65.625, 74.8) -> (-62.625, 74.8)
  line L63 (-62.625, 74.8) -> (-62.625, 72.8)
  line L64 (-62.625, 72.8) -> (-65.625, 72.8)
  line L65 (-65.625, 72.8) -> (-65.625, 74.8)
  line L66 (-41.25, 80.8) -> (-44.25, 80.8) projected
  line L67 (-44.25, 80.8) -> (-41.25, 80.8)
  line L68 (-41.25, 80.8) -> (-41.25, 82.8)
  line L69 (-41.25, 82.8) -> (-44.25, 82.8)
  line L70 (-44.25, 82.8) -> (-44.25, 80.8)
  line L71 (-44.25, 80.8) -> (-44.25, 74.8) projected
  line L72 (-44.25, 74.8) -> (-41.25, 74.8)
  line L73 (-41.25, 74.8) -> (-41.25, 72.8)
  line L74 (-41.25, 72.8) -> (-44.25, 72.8)
  line L75 (-44.25, 72.8) -> (-44.25, 74.8)
  line L76 (-19.875, 80.8) -> (-22.875, 80.8) projected
  line L77 (-22.875, 80.8) -> (-19.875, 80.8)
  line L78 (-19.875, 80.8) -> (-19.875, 82.8)
  line L79 (-19.875, 82.8) -> (-22.875, 82.8)
  line L80 (-22.875, 82.8) -> (-22.875, 80.8)
  line L81 (-22.875, 74.8) -> (-19.875, 74.8) projected
  line L82 (-22.875, 74.8) -> (-19.875, 74.8)
  line L83 (-19.875, 74.8) -> (-19.875, 72.8)
  line L84 (-19.875, 72.8) -> (-22.875, 72.8)
  line L85 (-22.875, 72.8) -> (-22.875, 74.8)
  line L86 (-62.625, 60.8) -> (-65.625, 60.8) projected
  line L87 (-65.625, 60.8) -> (-62.625, 60.8)
  line L88 (-62.625, 60.8) -> (-62.625, 62.8)
  line L89 (-62.625, 62.8) -> (-65.625, 62.8)
  line L90 (-65.625, 62.8) -> (-65.625, 60.8)
  line L91 (-65.625, 54.8) -> (-65.625, 60.8) projected
  line L92 (-65.625, 54.8) -> (-62.625, 54.8)
  line L93 (-62.625, 54.8) -> (-62.625, 52.8)
  line L94 (-62.625, 52.8) -> (-65.625, 52.8)
  line L95 (-65.625, 52.8) -> (-65.625, 54.8)
  line L96 (-62.625, 40.8) -> (-65.625, 40.8) projected
  line L97 (-65.625, 40.8) -> (-62.625, 40.8)
  line L98 (-62.625, 40.8) -> (-62.625, 42.8)
  line L99 (-62.625, 42.8) -> (-65.625, 42.8)
  line L100 (-65.625, 42.8) -> (-65.625, 40.8)
  line L101 (-65.625, 34.8) -> (-62.625, 34.8) projected
  line L102 (-65.625, 34.8) -> (-62.625, 34.8)
  line L103 (-62.625, 34.8) -> (-62.625, 32.8)
  line L104 (-62.625, 32.8) -> (-65.625, 32.8)
  line L105 (-65.625, 32.8) -> (-65.625, 34.8)
  line L106 (-65.625, 20.8) -> (-62.625, 20.8)
  line L107 (-62.625, 20.8) -> (-62.625, 22.8)
  line L108 (-62.625, 22.8) -> (-65.625, 22.8)
  line L109 (-65.625, 22.8) -> (-65.625, 20.8)
  line L110 (-65.625, 14.8) -> (-62.625, 14.8) projected
  line L111 (-65.625, 14.8) -> (-62.625, 14.8)
  line L112 (-62.625, 14.8) -> (-62.625, 12.8)
  line L113 (-62.625, 12.8) -> (-65.625, 12.8)
  line L114 (-65.625, 12.8) -> (-65.625, 14.8)
  line L115 (-44.25, 54.8) -> (-44.25, 60.8) projected
  line L116 (-44.25, 60.8) -> (-41.25, 60.8)
  line L117 (-41.25, 60.8) -> (-41.25, 62.8)
  line L118 (-41.25, 62.8) -> (-44.25, 62.8)
  line L119 (-44.25, 62.8) -> (-44.25, 60.8)
  line L120 (-41.25, 54.8) -> (-44.25, 54.8) projected
  line L121 (-44.25, 54.8) -> (-41.25, 54.8)
  line L122 (-41.25, 54.8) -> (-41.25, 52.8)
  line L123 (-41.25, 52.8) -> (-44.25, 52.8)
  line L124 (-44.25, 52.8) -> (-44.25, 54.8)
  line L125 (-19.875, 60.8) -> (-22.875, 60.8) projected
  line L126 (-22.875, 60.8) -> (-19.875, 60.8)
  line L127 (-19.875, 60.8) -> (-19.875, 62.8)
  line L128 (-19.875, 62.8) -> (-22.875, 62.8)
  line L129 (-22.875, 62.8) -> (-22.875, 60.8)
  line L130 (-19.875, 54.8) -> (-22.875, 54.8) projected
  line L131 (-22.875, 54.8) -> (-19.875, 54.8)
  line L132 (-19.875, 54.8) -> (-19.875, 52.8)
  line L133 (-19.875, 52.8) -> (-22.875, 52.8)
  line L134 (-22.875, 52.8) -> (-22.875, 54.8)
  line L135 (-44.25, 40.8) -> (-41.25, 40.8) projected
  line L136 (-44.25, 40.8) -> (-41.25, 40.8)
  line L137 (-41.25, 40.8) -> (-41.25, 42.8)
  line L138 (-41.25, 42.8) -> (-44.25, 42.8)
  line L139 (-44.25, 42.8) -> (-44.25, 40.8)
  line L140 (-44.25, 34.8) -> (-41.25, 34.8)
  line L141 (-41.25, 34.8) -> (-41.25, 32.8)
  line L142 (-41.25, 32.8) -> (-44.25, 32.8)
  line L143 (-44.25, 32.8) -> (-44.25, 34.8)
  line L144 (-44.25, 20.8) -> (-44.25, 14.8) projected
  line L145 (-44.25, 20.8) -> (-41.25, 20.8)
  line L146 (-41.25, 20.8) -> (-41.25, 22.8)
  line L147 (-41.25, 22.8) -> (-44.25, 22.8)
  line L148 (-44.25, 22.8) -> (-44.25, 20.8)
  line L149 (-44.25, 14.8) -> (-41.25, 14.8)
  line L150 (-41.25, 14.8) -> (-41.25, 12.8)
  line L151 (-41.25, 12.8) -> (-44.25, 12.8)
  line L152 (-44.25, 12.8) -> (-44.25, 14.8)
  line L153 (-22.875, 20.8) -> (-22.875, 14.8) projected
  line L154 (-22.875, 20.8) -> (-19.875, 20.8)
  line L155 (-19.875, 20.8) -> (-19.875, 22.8)
  line L156 (-19.875, 22.8) -> (-22.875, 22.8)
  line L157 (-22.875, 22.8) -> (-22.875, 20.8)
  line L158 (-22.875, 14.8) -> (-19.875, 14.8)
  line L159 (-19.875, 14.8) -> (-19.875, 12.8)
  line L160 (-19.875, 12.8) -> (-22.875, 12.8)
  line L161 (-22.875, 12.8) -> (-22.875, 14.8)
  line L162 (-22.875, 40.8) -> (-19.875, 40.8)
  line L163 (-19.875, 40.8) -> (-19.875, 42.8)
  line L164 (-19.875, 42.8) -> (-22.875, 42.8)
  line L165 (-22.875, 42.8) -> (-22.875, 40.8)
  line L166 (-22.875, 34.8) -> (-19.875, 34.8)
  line L167 (-19.875, 34.8) -> (-19.875, 32.8)
  line L168 (-19.875, 32.8) -> (-22.875, 32.8)
  line L169 (-22.875, 32.8) -> (-22.875, 34.8)
  point P0 (0, 0)
  dimension "d144" = 3
  dimension "d145" = 2
  dimension "d146" = 3
  dimension "d147" = 2
  dimension "d148" = 2
  dimension "d149" = 2
  dimension "d150" = 2
  dimension "d151" = 2
  dimension "d152" = 2
  dimension "d153" = 2
  dimension "d154" = 2
  dimension "d155" = 3
  dimension "d156" = 2
  dimension "d157" = 2
  dimension "d158" = 2
  dimension "d159" = 2
  dimension "d160" = 2
  constraints: 288 end point, 72 parallel, 43 point on line, 36 horizontal, 36 perpendicular
  measures "d144" distance of L3.end L2.end
  measures "d145" distance of L2.end L1.end
  measures "d146" distance of L7.end L8.end
  measures "d147" distance of L6.end L7.end
  measures "d148" distance of L31.end L30.end
  measures "d149" distance of L35.end L36.end
  measures "d150" distance of L59.end L58.end
  measures "d151" distance of L62.end L63.end
  measures "d152" distance of L68.end L67.end
  measures "d153" distance of L88.end L87.end
  measures "d154" distance of L92.end L93.end
  measures "d155" distance of L99.end L98.end
  measures "d156" distance of L98.end L97.end
  measures "d157" distance of L102.end L103.end
  measures "d158" distance of L107.end L106.end
  measures "d159" distance of L111.end L112.end
  measures "d160" distance of L117.end L116.end
extrude "Extrusion32" cut sketch "Sketch33" against normal blind 100
chamfer "Chamfer3" distance 5 angle 45 72 edges at (-62.625, 15, -117.8) (-62.625, 15, -97.8) (-62.625, 15, -77.8) (-62.625, 15, -57.8) (-62.625, 15, -37.8) (-62.625, 15, -17.8) (-65.625, 15, -117.8) (-65.625, 15, -97.8) (-65.625, 15, -77.8) (-65.625, 15, -57.8) (-65.625, 15, -37.8) (-65.625, 15, -17.8) (-44.25, 15, -117.8) (-44.25, 15, -97.8) (-44.25, 15, -77.8) (-44.25, 15, -57.8) (-44.25, 15, -37.8) (-44.25, 15, -17.8) (-41.25, 15, -117.8) (-41.25, 15, -97.8) (-41.25, 15, -77.8) (-41.25, 15, -57.8) (-41.25, 15, -37.8) (-41.25, 15, -17.8) (-22.875, 15, -117.8) (-22.875, 15, -97.8) (-22.875, 15, -77.8) (-22.875, 15, -57.8) (-22.875, 15, -37.8) (-22.875, 15, -17.8) (-19.875, 15, -117.8) (-19.875, 15, -97.8) (-19.875, 15, -77.8) (-19.875, 15, -57.8) (-19.875, 15, -37.8) (-19.875, 15, -17.8) (-64.125, 15, -22.8) (-64.125, 15, -12.8) (-42.75, 15, -22.8) (-42.75, 15, -12.8) (-64.125, 15, -32.8) (-64.125, 15, -42.8) (-64.125, 15, -52.8) (-42.75, 15, -32.8) (-42.75, 15, -42.8) (-42.75, 15, -62.8) (-64.125, 15, -62.8) (-42.75, 15, -52.8) (-21.375, 15, -42.8) (-21.375, 15, -22.8) (-21.375, 15, -12.8) (-21.375, 15, -32.8) (-21.375, 15, -62.8) (-21.375, 15, -52.8) (-21.375, 15, -82.8) (-21.375, 15, -72.8) (-42.75, 15, -82.8) (-42.75, 15, -72.8) (-64.125, 15, -82.8) (-64.125, 15, -72.8) (-64.125, 15, -92.8) (-64.125, 15, -102.8) (-64.125, 15, -112.8) (-64.125, 15, -122.8) (-42.75, 15, -122.8) (-42.75, 15, -112.8) (-42.75, 15, -102.8) (-42.75, 15, -92.8) (-21.375, 15, -92.8) (-21.375, 15, -102.8) (-21.375, 15, -112.8) (-21.375, 15, -122.8)
sketch "Sketch34" plane through (0, 15, 0) normal (0, 1, 0) x (1, 0, 0)
  point P0 (0, 0)
sketch "Sketch35" plane through (0, 15, 0) normal (0, 1, 0) x (1, 0, 0)
  line L0 (-75.5, 131.7) -> (-75.5, 3.9) projected
  line L1 (0, 3.9) -> (-10, 3.9) projected
  line L2 (-75.5, 131.7) -> (-10, 131.7)
  line L3 (-10, 131.7) -> (-10, 3.9)
  line L4 (-10, 3.9) -> (-75.5, 3.9)
  line L5 (-75.5, 3.9) -> (-75.5, 131.7)
  point P0 (0, 0)
  constraints: 8 end point, 2 parallel, 1 horizontal, 1 perpendicular
extrude "Extrusion33" add sketch "Sketch35" against normal blind 15
sketch "Sketch36" plane through (0, 15, 0) normal (0, 1, 0) x (1, 0, 0)
  line L0 (-10, 3.9) -> (-10, 131.7) projected
  line L1 (-10, 67.8) -> (-75.5, 67.8)
  line L2 (-75.5, 131.7) -> (-75.5, 3.9) projected
  line L3 (-75.5, 3.9) -> (-10, 3.9) projected
  line L4 (-42.75, 3.9) -> (-42.75, 67.8)
  line L5 (-42.75, 67.8) -> (-42.75, 131.7)
  line L6 (-75.5, 131.7) -> (-10, 131.7) projected
  circle A0 centre (-42.75, 99.75) radius 25.4
  circle A1 centre (-42.75, 35.85) radius 25.4
  point P0 (0, 0)
  dimension "d168" = 50.8
  dimension "d169" = 50.8
  constraints: 7 midpoint, 6 end point, 2 centre point
  measures "d168" diameter of A0
  measures "d169" diameter of A1
extrude "Extrusion34" cut sketch "Sketch36" against normal blind 15 contours A1 L4 | L4 A1 | A0 L5 | L5 A0
sketch "Sketch37" plane through (0, 15, 0) normal (0, 1, 0) x (1, 0, 0)
  circle A0 centre (-42.75, 99.75) radius 25.4 projected
  circle A1 centre (-42.75, 99.75) radius 27.9
  circle A2 centre (-42.75, 35.85) radius 25.4 projected
  circle A3 centre (-42.75, 35.85) radius 27.9
  line L0 (-10, 3.9) -> (-10, 131.7) projected
  line L1 (-75.5, 131.7) -> (-75.5, 3.9) projected
  line L2 (-10, 131.7) -> (-75.5, 131.7)
  line L3 (-75.5, 131.7) -> (-75.5, 3.9)
  line L4 (-75.5, 3.9) -> (-10, 3.9)
  line L5 (-10, 3.9) -> (-10, 131.7)
  point P0 (0, 0)
  dimension "d172" = 55.8
  dimension "d173" = 55.8
  constraints: 8 end point, 2 centre point, 2 coincident, 2 parallel, 1 horizontal, 1 perpendicular
  measures "d172" diameter of A1
  measures "d173" diameter of A3
extrude "Extrusion35" cut sketch "Sketch37" against normal blind 10 contours L4 L1 L2 L0
body "Solid1"
